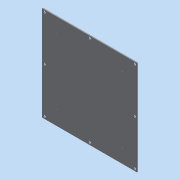
# Autodesk Inventor part: bed plate square
Saved by Autodesk Inventor 2015 (Build 190159000, 159)
## iProperties
Created: 2016-06-24
Part Number: bed plate square
Material: Generic
Document SubType Name: Modeling
Designer: Dustin
Density: 1 g/cm^3
Appearance: Default
Author: Dustin
Autodesk Inventor part; units mm, degrees
ref_plane "YZ Plane" through (0, 0, 0) normal (1, 0, 0) x (0, 1, 0)
ref_plane "XZ Plane" through (0, 0, 0) normal (0, 1, 0) x (-1, 0, 0)
ref_plane "XY Plane" through (0, 0, 0) normal (0, 0, 1) x (1, 0, 0)
sketch "Sketch1" plane through (0, 0, 0) normal (0, 0, 1) x (1, 0, 0)
  line L0 (0, 0) -> (300, 0)
  line L1 (300, 0) -> (300, 300)
  line L2 (300, 300) -> (0, 300)
  line L3 (0, 300) -> (0, 0)
  dimension "d0" = 300
  dimension "d1" = 300
  constraints: 8 end point, 2 parallel, 1 horizontal, 1 perpendicular
  measures "d0" distance of L2.end L0.start
  measures "d1" distance of L0.start L0.end
extrude "Extrusion1" add sketch "Sketch1" along normal blind 3.175
sketch "Sketch2" plane through (0, 0, 3.175) normal (0, 0, 1) x (1, 0, 0)
  line L0 (0, 300) -> (0, 0) projected
  line L1 (300, 300) -> (0, 300) projected
  line L2 (300, 0) -> (300, 300) projected
  line L3 (0, 0) -> (300, 0) projected
  point P0 (7, 293)
  point P1 (293, 293)
  point P2 (293, 7)
  point P3 (7, 7)
  dimension "d4" = 7
  dimension "d5" = 7
  dimension "d6" = 7
  dimension "d7" = 7
  dimension "d8" = 7
  dimension "d9" = 7
  dimension "d10" = 7
  dimension "d11" = 7
  measures "d4" distance from line of L0 point (7, 293)
  measures "d5" distance from line of L1 point (7, 293)
  measures "d6" distance from line of L2 point (293, 293)
  measures "d7" distance from line of L1 point (293, 293)
  measures "d8" distance from line of point (293, 7) L2
  measures "d9" distance from line of L3 point (293, 7)
  measures "d10" distance from line of L0 point (7, 7)
  measures "d11" distance from line of L3 point (7, 7)
hole "Hole1" at (7, 293, 3.175) at (293, 293, 3.175) at (293, 7, 3.175) at (7, 7, 3.175) direction (0, 0, -1) diameter 8 depth 25.4 tip angle 118
sketch "Sketch3" plane through (0, 0, 3.175) normal (0, 0, 1) x (1, 0, 0)
  line L0 (0, 300) -> (0, 0) projected
  line L1 (0, 0) -> (300, 0) projected
  line L2 (300, 0) -> (300, 300) projected
  point P0 (46, 254)
  point P1 (254, 254)
  point P2 (254, 46)
  point P3 (46, 46)
  dimension "d19" = 208
  dimension "d20" = 208
  dimension "d21" = 208
  dimension "d22" = 46
  dimension "d23" = 46
  dimension "d24" = 46
  dimension "d25" = 208
  dimension "d26" = 46
  measures "d19" distance of point (254, 254) point (46, 254)
  measures "d20" distance of point (46, 254) point (46, 46)
  measures "d21" distance of point (46, 46) point (254, 46)
  measures "d22" distance from line of L0 point (46, 46)
  measures "d23" distance from line of L1 point (46, 46)
  measures "d24" distance from line of L1 point (254, 46)
  measures "d25" distance of point (254, 46) point (254, 254)
  measures "d26" distance from line of L2 point (254, 254)
hole "Hole2" at (46, 254, 3.175) at (254, 254, 3.175) at (254, 46, 3.175) at (46, 46, 3.175) direction (0, 0, -1) diameter 3 depth 25.4 tip angle 118
sketch "Sketch4" plane through (0, 0, 3.175) normal (0, 0, 1) x (1, 0, 0)
  line L0 (0, 0) -> (300, 0) projected
  line L1 (0, 300) -> (0, 0) projected
  line L2 (300, 0) -> (300, 300) projected
  line L3 (300, 300) -> (0, 300) projected
  point P0 (150, 7)
  point P1 (293, 150)
  point P2 (150, 293)
  point P3 (7, 150)
  dimension "d34" = 150
  dimension "d35" = 7
  dimension "d36" = 7
  dimension "d37" = 150
  dimension "d38" = 7
  dimension "d39" = 7
  dimension "d40" = 150
  dimension "d41" = 150
  measures "d34" distance from line of L0 point (7, 150)
  measures "d35" distance from line of L1 point (7, 150)
  measures "d36" distance from line of L0 point (150, 7)
  measures "d37" distance from line of L2 point (150, 7)
  measures "d38" distance from line of L2 point (293, 150)
  measures "d39" distance from line of L3 point (150, 293)
  measures "d40" distance from line of L2 point (150, 293)
  measures "d41" distance from line of L0 point (293, 150)
hole "Hole3" at (150, 7, 3.175) at (293, 150, 3.175) at (150, 293, 3.175) at (7, 150, 3.175) direction (0, 0, -1) diameter 8 depth 25.4 tip angle 118
body "Solid1"
